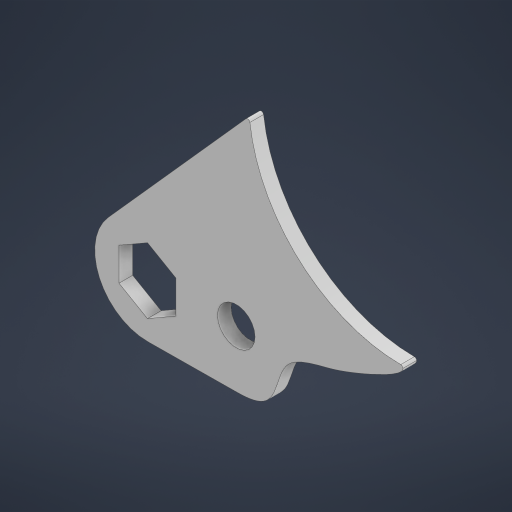
# Autodesk Inventor part: gear-interface-v3
Saved by Autodesk Inventor 2023.2 (Build 272271000, 271)
## iProperties
Created: 2023-03-26
Part Number: gear-interface-v3
Material: Generic
Document SubType Name: Modeling
Designer: Liam
Density: 1 g/cm^3
Appearance: Default
Author: Liam
Autodesk Inventor part; units mm, degrees
ref_plane "YZ Plane" through (0, 0, 0) normal (1, 0, 0) x (0, 1, 0)
ref_plane "XZ Plane" through (0, 0, 0) normal (0, 1, 0) x (-1, 0, 0)
ref_plane "XY Plane" through (0, 0, 0) normal (0, 0, 1) x (1, 0, 0)
sketch "Sketch1" plane through (0, 0, 0) normal (0, 0, 1) x (1, 0, 0)
  line L0 (-13.08, 1.2699) -> (-13.08, -2.3962)
  line L1 (-13.08, -2.3962) -> (-9.905, -4.2293)
  line L2 (-9.905, -4.2293) -> (-6.73, -2.3962)
  line L3 (-6.73, -2.3962) -> (-6.73, 1.2699)
  line L4 (-6.73, 1.2699) -> (-9.905, 3.103)
  line L5 (-9.905, 3.103) -> (-13.08, 1.2699)
  arc A0 (1.5178, 20.4301) -> (18.3452, 5.4526) centre (18.4703, 22.5348) ccw
  line L6 (-9.8521, -6.4389) -> (0.0571, -6.3497)
  arc A1 (-14.2892, 3.3491) -> (-9.8521, -6.4389) centre (-9.905, -0.5631) ccw
  arc A2 (1.5178, 20.4301) -> (1.0762, 20.5679) centre (1.2657, 20.3988) ccw
  arc A3 (18.5967, 5.2168) -> (18.3452, 5.4526) centre (18.3434, 5.1986) ccw
  circle A4 centre (0, 0) radius 2.0955
  line L7 (18.5967, 5.2168) -> (18.6555, 4.3986) construction
  line L8 (18.6555, 4.3986) -> (11.7907, 1.3579) construction
  line L9 (11.7907, 1.3579) -> (10.196, 1.1161) construction
  line L10 (10.196, 1.1161) -> (7.3568, 0.3252) construction
  line L11 (7.3568, 0.3252) -> (5.4578, -0.6554) construction
  line L12 (5.4578, -0.6554) -> (4.5551, -3.1132) construction
  line L13 (4.5551, -3.1132) -> (4.0373, -5.5547) construction
  line L14 (4.0373, -5.5547) -> (2.0974, -6.3497) construction
  line L15 (2.0974, -6.3497) -> (0.0571, -6.3497) construction
  spline S0 degree 4 poles (18.5967, 5.2168) (18.6555, 4.3986) (11.7907, 1.3579) (10.196, 1.1161) (7.3568, 0.3252) (5.4578, -0.6554) (4.5551, -3.1132) (4.0373, -5.5547) (2.0974, -6.3497) (0.0571, -6.3497) knots 1 1 1 1 1 2 3 4 5 6 7 7 7 7 7
  line L16 (-14.2892, 3.3491) -> (1.0762, 20.5679)
  point P0 (-9.9025, -0.563)
  point P1 (1.4887, 20.6794)
  point P2 (19.9848, 5.5194)
  dimension "d2" = 7.3323
  dimension "d3" = 7.3323
  dimension "d4" = 7.3323
  dimension "d12" = 0.254
  dimension "d13" = 3.6662
  dimension "d14" = 3.6662
  dimension "d15" = 4.191
  constraints: 16 end point, 10 point on circle, 5 centre point, 4 equal length, 4 tangent, 2 parallel, 1 equal radius, 1 horizontal, 1 vertical, 9 other
  measures "d2" distance of L2.end L0.start
  measures "d3" distance of L3.end L0.end
  measures "d4" distance of L1.end L4.end
  measures "d12" radius of A2
  measures "d13" distance of L4.end A1.centre
  measures "d14" distance of A1.centre L0.start
  measures "d15" diameter of A4
extrude "Extrusion3" add sketch "Sketch1" along normal blind 1.524
equation "\"d3\" = d2"
equation "\"d4\" = d2"
equation "\"d13\" = 0.5 * d2"
equation "\"d14\" = 0.5 * d2"
body "Solid3"
